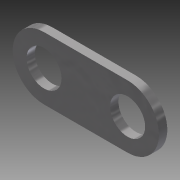
# Autodesk Inventor part: Solder Joint
Saved by Autodesk Inventor 2015 (Build 190159000, 159)
## iProperties
Created: 2016-01-20
Part Number: Solder Joint
Material: Generic
Document SubType Name: Modeling
Designer: Kyle
Density: 1 g/cm^3
Appearance: Galvanized
Author: Kyle
Autodesk Inventor part; units mm, degrees
ref_plane "YZ Plane" through (0, 0, 0) normal (1, 0, 0) x (0, 1, 0)
ref_plane "XZ Plane" through (0, 0, 0) normal (0, 1, 0) x (-1, 0, 0)
ref_plane "XY Plane" through (0, 0, 0) normal (0, 0, 1) x (1, 0, 0)
sketch "Sketch1" plane through (0, 0, 0) normal (0, 0, 1) x (1, 0, 0)
  line L0 (0, 0) -> (4.445, 0)
  line L1 (4.445, 0) -> (4.445, 1.905)
  line L2 (4.445, 1.905) -> (0, 1.905)
  line L3 (0, 1.905) -> (0, 0)
  circle A0 centre (0.9525, 0.9525) radius 0.5334
  circle A1 centre (3.4925, 0.9525) radius 0.5334
  dimension "d0" = 4.445
  dimension "d1" = 1.905
  dimension "d2" = 1.0668
  dimension "d3" = 0.9525
  dimension "d4" = 1.0668
  dimension "d5" = 2.54
  dimension "d6" = 0.9525
  constraints: 8 end point, 2 centre point, 2 parallel, 1 horizontal, 1 perpendicular
  measures "d0" distance of L1.end L2.end
  measures "d1" distance of L0.end L1.end
  measures "d2" diameter of A0
  measures "d3" distance from line of L0 A0.centre
  measures "d4" diameter of A1
  measures "d5" distance of A0.centre A1.centre
  measures "d6" distance from line of L1 A1.centre
extrude "Extrusion1" add sketch "Sketch1" along normal blind 0.254
fillet "Fillet1" radius 0.9525 4 edges at (4.445, 1.905, 0.127) (4.445, 0, 0.127) (0, 1.905, 0.127) (0, 0, 0.127)
body "Solid1"
